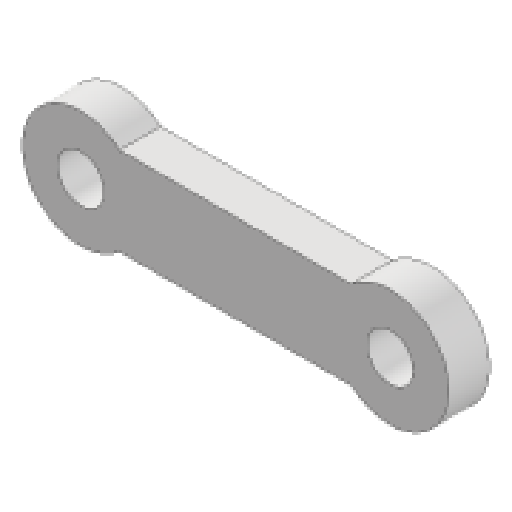
# Autodesk Inventor part: Arm 3
Saved by Autodesk Inventor 2025 (Build 290162010, 162A)
## iProperties
Created: 2024-11-29
Part Number: Arm 3
Material: Generic
Document SubType Name: Modeling
Designer: alexa
Density: 1 g/cm^3
Appearance: Default
Author: alexa
Autodesk Inventor part; units mm, degrees
ref_plane "YZ Plane" through (0, 0, 0) normal (1, 0, 0) x (0, 1, 0)
ref_plane "XZ Plane" through (0, 0, 0) normal (0, 1, 0) x (-1, 0, 0)
ref_plane "XY Plane" through (0, 0, 0) normal (0, 0, 1) x (1, 0, 0)
sketch "Sketch1" plane through (0, 0, 0) normal (0, 0, 1) x (1, 0, 0)
  arc A0 (3.3601, 3.81) -> (3.3601, -3.81) centre (0, 0) ccw
  circle A1 centre (0, 0) radius 2.032
  line L0 (3.3601, 3.81) -> (33.3683, 3.81)
  line L1 (3.3601, -3.81) -> (33.3683, -3.81)
  arc A2 (33.3683, -3.81) -> (33.3683, 3.81) centre (36.7284, 0) ccw
  circle A3 centre (36.7284, 0) radius 2.032
  dimension "d0" = 10.16
  dimension "d1" = 4.064
  dimension "d2" = 7.62
  dimension "d3" = 3.81
  dimension "d4" = 10.16
  dimension "d5" = 4.064
  dimension "d6" = 36.7284
  constraints: 4 centre point, 4 end point, 4 point on circle, 3 coincident, 2 horizontal, 1 horizontal alignment
  measures "d0" diameter of A0
  measures "d1" diameter of A1
  measures "d2" distance between parallel lines of L0 L1
  measures "d3" distance from line of point (0, 0) L0
  measures "d4" diameter of A2
  measures "d5" diameter of A3
  measures "d6" distance of A2.centre point (0, 0)
extrude "Extrusion1" add sketch "Sketch1" along normal blind 3.556
equation "\"d5\" = d1"
body "Solid1"
